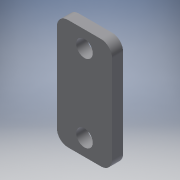
# Autodesk Inventor part: Cable_clamp
Saved by Autodesk Inventor 2019.3 (Build 233278000, 278)
## iProperties
Created: 2020-08-31
Part Number: Cable_clamp
Material: Generisch
Document SubType Name: Modeling
Designer: Nicolas Frick
Density: 1 g/cm^3
Appearance: Vorgabe
Author: Nicolas Frick
Autodesk Inventor part; units mm, degrees
ref_plane "YZ Plane" through (0, 0, 0) normal (1, 0, 0) x (0, 1, 0)
ref_plane "XZ Plane" through (0, 0, 0) normal (0, 1, 0) x (-1, 0, 0)
ref_plane "XY Plane" through (0, 0, 0) normal (0, 0, 1) x (1, 0, 0)
sketch "Skizze1" plane through (0, 0, 0) normal (0, 0, 1) x (1, 0, 0)
  circle A0 centre (0, -7.0156) radius 1.25 construction
  line L0 (-5, -4.0311) -> (5, -4.0311) construction
  line L1 (-5, -4.0311) -> (-5, -10) construction
  line L2 (-5, -10) -> (5, -10) construction
  line L3 (5, -10) -> (5, -4.0311) construction
  circle A1 centre (0, 7.0156) radius 1.25 construction
  line L4 (5, 4.0311) -> (-5, 4.0311) construction
  line L5 (5, 4.0311) -> (5, 10) construction
  line L6 (5, 10) -> (-5, 10) construction
  line L7 (-5, 10) -> (-5, 4.0311) construction
  line L8 (5, 10) -> (-5, 10)
  line L9 (-5, 10) -> (-5, -10)
  line L10 (-5, -10) -> (5, -10)
  line L11 (5, -10) -> (5, 10)
  circle A2 centre (0, 7.0156) radius 1.5
  circle A3 centre (0, -7.0156) radius 1.5
  point P0 (0, 0)
  dimension "d0" = 3
  dimension "d1" = 3
  constraints: 8 end point, 2 centre point, 2 coincident, 2 parallel, 1 horizontal, 1 perpendicular
  measures "d0" diameter of A2
  measures "d1" diameter of A3
extrude "Extrusion1" add sketch "Skizze1" along normal blind 2
fillet "Rundung1" radius 2 4 edges at (5, 10, 1) (-5, 10, 1) (-5, -10, 1) (5, -10, 1)
